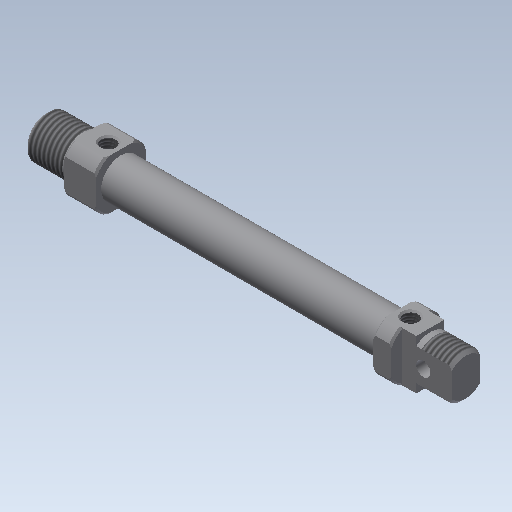
# Autodesk Inventor part: RM/8010/M/50_B0__B
Saved by Autodesk Inventor 2020.5 (Build 245400000, 400)
## iProperties
Created: 2018-09-27
Part Number: RM/8010/M/50_B0__B
Material: Generic
Catalog Web Link: www.cadenas.de
Description: Series RM/8000/M BODY-ISO Cylinder
Vendor: IMI
Document SubType Name: Modeling
Designer: psadmin
Manufacturer: IMI
Mass: 6.11962 g
Surface Area: 79.4353 cm^2
Volume: 6.11962 cm^3
Density: 1 g/cm^3
Appearance: PSOLRGB-192-192-192
Category: PARTsolutions
Company: IMI
PSOL_IDENT_0: {$CADENAS_DATA\23d-libs\imi_precision\1_actuators\1_roundline_cylinders\parts\series_rm_8000_m_body.
PSOL_IDENT_1: prj},233 {VTYP=3D},{NB=RM/8010/M/50_B0__B},{LINA=RM/8010/M/50_B0__B},{NN=Series RM/8000/M BODY},{DAT
PSOL_IDENT_2: E=04.09.2018 05:58:30},{GEOMDATE=13.09.2016 07:04:00},{VERSION=},{LINEID=10},{WBVAR=CH,BS,HUB,HRS,VA
PSOL_IDENT_3: R,PMU,PR,FM,LMT,RMT},{WBNUMERIC=HUB,PMU}  {NB=RM/8010/M/50_B0__B},{LINA=RM/8010/M/50_B0__B},{KT=DUMM
PSOL_IDENT_4: Y},{CNSORDERNO=RM/8010/M/50},{CH=B},{BS=010},{DALG=  '010' , '10' ,  '012' , '12'  ,  '016' , '16' ,
PSOL_IDENT_5: '020' , '20' ,  '025' , '25'  },{HUB=50},{HUBALG=[0:500/1]},{HRS=},{HRSALG= '' ,  'Standard (pneum
PSOL_IDENT_6: atic)'  },{P=Magnetic Piston},{VAR=M},{VARALG=    'M' , 'M - Standard with integral eye mounting, no
PSOL_IDENT_7: variant' ,  'MC' , 'MC - Central rear port' ,  'MF' , 'MF - Flat rear cover'  , 'MU' , 'MU - Extend
PSOL_IDENT_8: ed piston rod'    },{PMU=0},{PMUALG=0},{PR=},{PRALG= '' , 'None' , '+QM/8010/38' , 'AK - Piston rod
PSOL_IDENT_9: swivel' , '+QM/8010/25' , 'F - Piston rod clevis' , '+QM/8010/32' , 'UF - Piston rod eye' },{FM=},{F
PSOL_IDENT_10: MALG= '' , 'None' , '+M/P19369' , 'C - Foot Mounting' , '+M/P19407' , 'B/G - Front/rear flange'  },{
PSOL_IDENT_11: LMT=},{LMTALG= '' , 'None' , '+M/P19369' , 'C - Foot Mounting' , '+M/P19407' , 'B/G - Front/rear fla
PSOL_IDENT_12: nge'  },{RMT=},{RMTALG= '' , 'None' , '+M/P19369' , 'C - Foot Mounting' , '+M/P19407' , 'B/G - Front
PSOL_IDENT_13: /rear flange'  },{AM=12},{B=12},{BA=12},{BE=M12x1.25},{BF=12},{CD=4},{D=16.5},{EE=M5},{EW=7.9},{G=9.
PSOL_IDENT_14: 0},{KK=M4},{KV=19},{KW=6},{KW1=2},{L=6},{L12=0},{LB=2},{MM=4},{MR=8},{PL=5.5},{KV1=7},{KV2=0},{KV4=1
PSOL_IDENT_15: 4},{WF=16},{VA=1.5},{VD=1.5},{XC=64},{BEX=12.000},{BEP=1.250},{EEX=5.000},{EEP=0.800},{KKX=4.000},{K
PSOL_IDENT_16: KP=0.700},{BSX=10},{BSY=11.100},{ANG=0.500},{DEEP=3.000},{L8=0},{ZM=0},{ZJ=62},{AD=0.0},{AC=10.000},
PSOL_IDENT_17: {XC2=0.000},{AD2=0},{WF2=0},{BF2=0},{MOVE=2.000},{XYZ=0},{FMMOVE=0.0},{MOVE61=0},{MOVE2=2},{MOVEL4=0
PSOL_IDENT_18: }
NN: Series RM/8000/M BODY
NT: ISO Cylinder
NB: RM/8010/M/50_B0__B
NBSYN: $CNSORDERNO._$CH.$PMU.$LMT._$RMT._B
LINA: RM/8010/M/50_B0__B
CNSORDERNO: RM/8010/M/50
CH: Buffer
BS: 10
HUB: 50
HRS: Standard (pneumatic)
VAR: M - Standard with integral eye mounting, no variant
PMU: 0
AM: 12
B: 12
BA: 12
BE: M12x1.25
BF: 12
CD: 4
D: 16.5
EE: M5
EW: 7.9
G: 9
KK: M4
KV: 19
KW: 6
KW1: 2
L: 6
L12: 0
LB: 2
MM: 4
MR: 8
PL: 5.5
WF: 16
VA: 1.5
VD: 1.5
XC: 64
SUPPLIER: IMI
ARTICLENO: RM/8010/M/50_B0__B
BOMINFO: RM/8010/M/50_B0__B
CREATOR: CADENAS GmbH
Title: RM/8010/M/50_B0__B
Author: Cadenas PARTsolutions
Comments: ISO Cylinder
Autodesk Inventor part; units mm, degrees
sketch "Sketch_2" plane through (0, 0, 0) normal (0, 0, 1) x (1, 0, 0)
  line L0 (106, 0) -> (-12, 0)
  line L1 (87, 0) -> (87, 5)
  line L2 (87, 5) -> (9, 5)
  line L3 (9, 5) -> (9, 2)
  line L4 (9, 2) -> (-12, 2)
  line L5 (-12, 2) -> (-12, 5.233)
  line L6 (-12, 5.233) -> (-11.233, 6)
  line L7 (-11.233, 6) -> (0, 6)
  line L8 (0, 6) -> (0, 7.75)
  line L9 (0, 7.75) -> (0.5, 8.25)
  line L10 (0.5, 8.25) -> (8.5, 8.25)
  line L11 (8.5, 8.25) -> (9, 7.75)
  line L12 (9, 7.75) -> (9, 5.55)
  line L13 (9, 5.55) -> (87, 5.55)
  line L14 (87, 5.55) -> (87, 7.75)
  line L15 (87, 7.75) -> (87.5, 8.25)
  line L16 (87.5, 8.25) -> (91.5, 8.25)
  line L17 (91.5, 8.25) -> (92, 7.75)
  line L18 (92, 7.75) -> (92, 6)
  line L19 (92, 6) -> (105.233, 6)
  line L20 (105.233, 6) -> (106, 5.233)
  line L21 (106, 5.233) -> (106, 0)
  line L22 (106, 0) -> (87, 0)
  constraints: 46 end point
revolve "Revolution1" add sketch "Sketch_2" angle 360 about axis through (106, 0, 0) along (1, 0, 0)
thread "Thread1" size "M12x1.25" class "6g" standard "ISO Metric profile" length 9.733
thread "Thread2" size "M12x1.25" class "6g" standard "ISO Metric profile" length 7.733
sketch "Sketch_3" plane through (0, 0, 0) normal (0, 1, 0) x (-1, 0, 0)
  line L0 (-87, 3.45) -> (-87.5, 3.95)
  line L1 (-87.5, 3.95) -> (-96, 3.95)
  line L2 (-96, 3.95) -> (-96, -3.95)
  line L3 (-96, -3.95) -> (-87.5, -3.95)
  line L4 (-87.5, -3.95) -> (-87, -3.45)
  line L5 (-87, -3.45) -> (-87, 3.45)
  constraints: 12 end point
extrude "Extrusion1" add sketch "Sketch_3" along normal mid plane 16.5
sketch "Sketch_4" plane through (0, 0, 0) normal (0, 1, 0) x (-1, 0, 0)
  line L0 (-92, 13.95) -> (-111, 13.95)
  line L1 (-111, 13.95) -> (-111, -13.95)
  line L2 (-111, -13.95) -> (-92, -13.95)
  line L3 (-92, -13.95) -> (-92, -3.95)
  line L4 (-92, -3.95) -> (-106, -3.95)
  line L5 (-106, -3.95) -> (-106, 3.95)
  line L6 (-106, 3.95) -> (-92, 3.95)
  line L7 (-92, 3.95) -> (-92, 13.95)
  constraints: 16 end point
extrude "Extrusion2" cut sketch "Sketch_4" along normal mid plane 16.5
sketch "Sketch_5" plane through (0, 0, 0) normal (1, 0, 0) x (0, 1, 0)
  line L0 (-14, 14) -> (-14, -14)
  line L1 (-14, -14) -> (14, -14)
  line L2 (14, -14) -> (14, 14)
  line L3 (14, 14) -> (-14, 14)
  line L4 (-7, 7) -> (-7, -7)
  line L5 (-7, -7) -> (7, -7)
  line L6 (7, -7) -> (7, 7)
  line L7 (7, 7) -> (-7, 7)
  constraints: 16 end point
extrude "Extrusion3" cut sketch "Sketch_5" along normal blind 9
sketch "Sketch_6" plane through (90.5, 0, 0) normal (1, 0, 0) x (0, 0, -1)
  line L0 (-14, -14) -> (14, -14)
  line L1 (14, -14) -> (14, 14)
  line L2 (14, 14) -> (-14, 14)
  line L3 (-14, 14) -> (-14, -14)
  line L4 (-7, -7) -> (7, -7)
  line L5 (7, -7) -> (7, 7)
  line L6 (7, 7) -> (-7, 7)
  line L7 (-7, 7) -> (-7, -7)
  constraints: 16 end point
extrude "Extrusion4" cut sketch "Sketch_6" along normal mid plane 18
sketch "Sketch6" plane through (0.5, 7, -4.3661) normal (0, 1, 0) x (1, 0, 0)
  point P0 (5, -4.3661)
hole "Hole1" at (5.5, 7, 0) direction (0, -1, 0) diameter 4.134 depth 7 countersink diameter 5 countersink angle 90 thread size "M5x0.8" class "6H" standard "ISO Metric profile"
sketch "Sketch7" plane through (91.7124, 7, 3.95) normal (0, 1, 0) x (1, 0, 0)
  point P0 (-1.2124, 3.95)
hole "Hole2" at (90.5, 7, 0) direction (0, -1, 0) diameter 4.134 depth 7 countersink diameter 5 countersink angle 90 thread size "M5x0.8" class "6H" standard "ISO Metric profile"
sketch "Sketch_9" plane through (0, 0, 0) normal (0, 0, 1) x (1, 0, 0)
  circle A0 centre (98, 0) radius 2
  constraints: 1 centre point
extrude "Extrusion5" cut sketch "Sketch_9" along normal mid plane 7.9
ref_plane "AC_XY" through (98, 0, 0) normal (0, 0, 1) x (1, 0, 0)
ref_plane "AC_YZ" through (98, 0, 0) normal (1, 0, 0) x (0, 1, 0)
ref_plane "AC_ZX" through (98, 0, 0) normal (0, 1, 0) x (0, 0, 1)
ref_plane "DUMMY_XY" through (0, 0, 0) normal (0, 1, 0) x (1, 0, 0)
ref_plane "DUMMY_YZ" through (0, 0, 0) normal (1, 0, 0) x (0, 0, -1)
ref_plane "DUMMY_ZX" through (0, 0, 0) normal (0, 0, -1) x (0, 1, 0)
ref_plane "FM_XY" through (0, 0, 0) normal (-1, 0, 0) x (0, 0, -1)
ref_plane "FM_YZ" through (0, 0, 0) normal (0, 0, -1) x (0, -1, 0)
ref_plane "FM_ZX" through (0, 0, 0) normal (0, -1, 0) x (-1, 0, 0)
ref_plane "FMFM_XY" through (0, 0, 0) normal (-1, 0, 0) x (0, 0, -1)
ref_plane "FMFM_YZ" through (0, 0, 0) normal (0, 0, -1) x (0, -1, 0)
ref_plane "FMFM_ZX" through (0, 0, 0) normal (0, -1, 0) x (-1, 0, 0)
ref_plane "NUT_XY" through (-2, 0, 0) normal (-1, 0, 0) x (0, 0, -1)
ref_plane "NUT_YZ" through (-2, 0, 0) normal (0, 0, -1) x (0, -1, 0)
ref_plane "NUT_ZX" through (-2, 0, 0) normal (0, -1, 0) x (-1, 0, 0)
ref_plane "POINT_XY" through (-12, 0, 0) normal (-1, 0, 0) x (0, 0, -1)
ref_plane "POINT_YZ" through (-12, 0, 0) normal (0, 0, -1) x (0, -1, 0)
ref_plane "POINT_ZX" through (-12, 0, 0) normal (0, -1, 0) x (-1, 0, 0)
ref_plane "RM_XY" through (96, 0, 0) normal (1, 0, 0) x (0, 0, -1)
ref_plane "RM_YZ" through (96, 0, 0) normal (0, 0, -1) x (0, 1, 0)
ref_plane "RM_ZX" through (96, 0, 0) normal (0, 1, 0) x (1, 0, 0)
ref_plane "S_XY" through (26, 0, 0) normal (1, 0, 0) x (0, 0, -1)
ref_plane "S_YZ" through (26, 0, 0) normal (0, 0, -1) x (0, 1, 0)
ref_plane "S_ZX" through (26, 0, 0) normal (0, 1, 0) x (1, 0, 0)
ref_plane "dim_0_XY" through (0, 0, 0) normal (0, 0, 1) x (1, 0, 0)
ref_plane "dim_0_YZ" through (0, 0, 0) normal (1, 0, 0) x (0, 1, 0)
ref_plane "dim_0_ZX" through (0, 0, 0) normal (0, 1, 0) x (0, 0, 1)
ref_plane "dim_bex1_XY" through (105.233, 6, 0) normal (0, 0, 1) x (1, 0, 0)
ref_plane "dim_bex1_YZ" through (105.233, 6, 0) normal (1, 0, 0) x (0, 1, 0)
ref_plane "dim_bex1_ZX" through (105.233, 6, 0) normal (0, 1, 0) x (0, 0, 1)
ref_plane "dim_bex2_XY" through (105.233, -6, 0) normal (0, 0, 1) x (1, 0, 0)
ref_plane "dim_bex2_YZ" through (105.233, -6, 0) normal (1, 0, 0) x (0, 1, 0)
ref_plane "dim_bex2_ZX" through (105.233, -6, 0) normal (0, 1, 0) x (0, 0, 1)
ref_plane "dim_cd1_XY" through (98, 2, 0) normal (0, 0, 1) x (1, 0, 0)
ref_plane "dim_cd1_YZ" through (98, 2, 0) normal (1, 0, 0) x (0, 1, 0)
ref_plane "dim_cd1_ZX" through (98, 2, 0) normal (0, 1, 0) x (0, 0, 1)
ref_plane "dim_cd2_XY" through (98, -2, 0) normal (0, 0, 1) x (1, 0, 0)
ref_plane "dim_cd2_YZ" through (98, -2, 0) normal (1, 0, 0) x (0, 1, 0)
ref_plane "dim_cd2_ZX" through (98, -2, 0) normal (0, 1, 0) x (0, 0, 1)
ref_plane "dim_d1_XY" through (18, 5.55, 0) normal (0, 0, 1) x (1, 0, 0)
ref_plane "dim_d1_YZ" through (18, 5.55, 0) normal (1, 0, 0) x (0, 1, 0)
ref_plane "dim_d1_ZX" through (18, 5.55, 0) normal (0, 1, 0) x (0, 0, 1)
ref_plane "dim_d2_XY" through (18, -5.55, 0) normal (0, 0, 1) x (1, 0, 0)
ref_plane "dim_d2_YZ" through (18, -5.55, 0) normal (1, 0, 0) x (0, 1, 0)
ref_plane "dim_d2_ZX" through (18, -5.55, 0) normal (0, 1, 0) x (0, 0, 1)
ref_plane "dim_ee_XY" through (5.5, 7, 0) normal (0, 0, 1) x (1, 0, 0)
ref_plane "dim_ee_YZ" through (5.5, 7, 0) normal (1, 0, 0) x (0, 1, 0)
ref_plane "dim_ee_ZX" through (5.5, 7, 0) normal (0, 1, 0) x (0, 0, 1)
ref_plane "dim_ee1_XY" through (3, 7, 0) normal (0, 0, 1) x (1, 0, 0)
ref_plane "dim_ee1_YZ" through (3, 7, 0) normal (1, 0, 0) x (0, 1, 0)
ref_plane "dim_ee1_ZX" through (3, 7, 0) normal (0, 1, 0) x (0, 0, 1)
ref_plane "dim_ee2_XY" through (8, 7, 0) normal (0, 0, 1) x (1, 0, 0)
ref_plane "dim_ee2_YZ" through (8, 7, 0) normal (1, 0, 0) x (0, 1, 0)
ref_plane "dim_ee2_ZX" through (8, 7, 0) normal (0, 1, 0) x (0, 0, 1)
ref_plane "dim_ew1_XY" through (96, 0, -3.95) normal (0, 1, 0) x (1, 0, 0)
ref_plane "dim_ew1_YZ" through (96, 0, -3.95) normal (1, 0, 0) x (0, 0, -1)
ref_plane "dim_ew1_ZX" through (96, 0, -3.95) normal (0, 0, -1) x (0, 1, 0)
ref_plane "dim_ew2_XY" through (96, 0, 3.95) normal (0, 1, 0) x (1, 0, 0)
ref_plane "dim_ew2_YZ" through (96, 0, 3.95) normal (1, 0, 0) x (0, 0, -1)
ref_plane "dim_ew2_ZX" through (96, 0, 3.95) normal (0, 0, -1) x (0, 1, 0)
ref_plane "dim_g_XY" through (9, 0, 0) normal (0, 0, 1) x (1, 0, 0)
ref_plane "dim_g_YZ" through (9, 0, 0) normal (1, 0, 0) x (0, 1, 0)
ref_plane "dim_g_ZX" through (9, 0, 0) normal (0, 1, 0) x (0, 0, 1)
ref_plane "dim_gew_bottom_XY" through (-12, -6, 0) normal (0, 0, 1) x (1, 0, 0)
ref_plane "dim_gew_bottom_YZ" through (-12, -6, 0) normal (1, 0, 0) x (0, 1, 0)
ref_plane "dim_gew_bottom_ZX" through (-12, -6, 0) normal (0, 1, 0) x (0, 0, 1)
ref_plane "dim_gew_top_XY" through (-12, 6, 0) normal (0, 0, 1) x (1, 0, 0)
ref_plane "dim_gew_top_YZ" through (-12, 6, 0) normal (1, 0, 0) x (0, 1, 0)
ref_plane "dim_gew_top_ZX" through (-12, 6, 0) normal (0, 1, 0) x (0, 0, 1)
ref_plane "dim_kv41_XY" through (0, 0, 7) normal (1, 0, 0) x (0, 0, -1)
ref_plane "dim_kv41_YZ" through (0, 0, 7) normal (0, 0, -1) x (0, 1, 0)
ref_plane "dim_kv41_ZX" through (0, 0, 7) normal (0, 1, 0) x (1, 0, 0)
ref_plane "dim_kv42_XY" through (0, 0, -7) normal (1, 0, 0) x (0, 0, -1)
ref_plane "dim_kv42_YZ" through (0, 0, -7) normal (0, 0, -1) x (0, 1, 0)
ref_plane "dim_kv42_ZX" through (0, 0, -7) normal (0, 1, 0) x (1, 0, 0)
ref_plane "dim_l_XY" through (92, 6, 0) normal (0, 0, 1) x (1, 0, 0)
ref_plane "dim_l_YZ" through (92, 6, 0) normal (1, 0, 0) x (0, 1, 0)
ref_plane "dim_l_ZX" through (92, 6, 0) normal (0, 1, 0) x (0, 0, 1)
ref_plane "dim_left_XY" through (-12, 0, 0) normal (0, 0, 1) x (1, 0, 0)
ref_plane "dim_left_YZ" through (-12, 0, 0) normal (1, 0, 0) x (0, 1, 0)
ref_plane "dim_left_ZX" through (-12, 0, 0) normal (0, 1, 0) x (0, 0, 1)
ref_plane "dim_right_XY" through (106, 0, 0) normal (0, 0, 1) x (1, 0, 0)
ref_plane "dim_right_YZ" through (106, 0, 0) normal (1, 0, 0) x (0, 1, 0)
ref_plane "dim_right_ZX" through (106, 0, 0) normal (0, 1, 0) x (0, 0, 1)
ref_plane "dim_right_g_XY" through (87, 0, 0) normal (0, 0, 1) x (1, 0, 0)
ref_plane "dim_right_g_YZ" through (87, 0, 0) normal (1, 0, 0) x (0, 1, 0)
ref_plane "dim_right_g_ZX" through (87, 0, 0) normal (0, 1, 0) x (0, 0, 1)
ref_plane "dim_right_hub_XY" through (96, 0, 0) normal (0, 0, 1) x (1, 0, 0)
ref_plane "dim_right_hub_YZ" through (96, 0, 0) normal (1, 0, 0) x (0, 1, 0)
ref_plane "dim_right_hub_ZX" through (96, 0, 0) normal (0, 1, 0) x (0, 0, 1)
ref_plane "dim_va_XY" through (97.5, 0, 0) normal (0, 0, 1) x (1, 0, 0)
ref_plane "dim_va_YZ" through (97.5, 0, 0) normal (1, 0, 0) x (0, 1, 0)
ref_plane "dim_va_ZX" through (97.5, 0, 0) normal (0, 1, 0) x (0, 0, 1)
body "Solid1"
